Autodesk Inventor part; units mm, degrees
(part 3 of 5)
sketch "Sketch5" plane through (0, 0, 5) normal (0, 0, 1) x (1, 0, 0)
  line L0 (140, 35) -> (-140, 35) projected
  line L1 (-140, -35) -> (140, -35) projected
  line L2 (-165, 10) -> (-165, -10) projected
  line L3 (165, -10) -> (165, 10) projected
  arc A0 (87.0071, 22.2929) -> (87.7142, 22) centre (87.7142, 23) ccw
  arc A1 (87.7142, 27) -> (87.0071, 26.7071) centre (87.7142, 26) ccw
  line L4 (87.0071, 22.2929) -> (85.1, 24.2)
  line L5 (87.0071, 26.7071) -> (85.1, 24.8)
  line L6 (85.1, 24.5) -> (85.1, 24.2)
  line L7 (85.1, 24.5) -> (85.1, 24.8)
  line L8 (87.7142, 27) -> (104.4858, 27)
  line L9 (104.4858, 22) -> (87.7142, 22)
  arc A2 (105.1929, 26.7071) -> (104.4858, 27) centre (104.4858, 26) ccw
  line L10 (105.1929, 26.7071) -> (107.1, 24.8)
  line L11 (107.1, 24.5) -> (107.1, 24.8)
  line L12 (107.1, 24.5) -> (107.1, 24.2)
  arc A3 (104.4858, 22) -> (105.1929, 22.2929) centre (104.4858, 23) ccw
  line L13 (105.1929, 22.2929) -> (107.1, 24.2)
  arc A4 (87.0071, -2.5071) -> (87.7142, -2.8) centre (87.7142, -1.8) ccw
  arc A5 (87.7142, 2.2) -> (87.0071, 1.9071) centre (87.7142, 1.2) ccw
  line L14 (87.0071, -2.5071) -> (85.1, -0.6)
  line L15 (87.0071, 1.9071) -> (85.1, 0)
  line L16 (85.1, -0.3) -> (85.1, -0.6)
  line L17 (85.1, -0.3) -> (85.1, 0)
  line L18 (87.7142, 2.2) -> (104.4858, 2.2)
  line L19 (104.4858, -2.8) -> (87.7142, -2.8)
  arc A6 (105.1929, 1.9071) -> (104.4858, 2.2) centre (104.4858, 1.2) ccw
  line L20 (105.1929, 1.9071) -> (107.1, 0)
  line L21 (107.1, -0.3) -> (107.1, 0)
  line L22 (107.1, -0.3) -> (107.1, -0.6)
  arc A7 (104.4858, -2.8) -> (105.1929, -2.5071) centre (104.4858, -1.8) ccw
  line L23 (105.1929, -2.5071) -> (107.1, -0.6)
  arc A8 (85.9071, 3.0071) -> (86.2, 3.7142) centre (85.2, 3.7142) ccw
  arc A9 (81.2, 3.7142) -> (81.4929, 3.0071) centre (82.2, 3.7142) ccw
  line L24 (85.9071, 3.0071) -> (84, 1.1)
  line L25 (81.4929, 3.0071) -> (83.4, 1.1)
  line L26 (83.7, 1.1) -> (84, 1.1)
  line L27 (83.7, 1.1) -> (83.4, 1.1)
  line L28 (81.2, 3.7142) -> (81.2, 20.4858)
  line L29 (86.2, 20.4858) -> (86.2, 3.7142)
  arc A10 (81.4929, 21.1929) -> (81.2, 20.4858) centre (82.2, 20.4858) ccw
  line L30 (81.4929, 21.1929) -> (83.4, 23.1)
  line L31 (83.7, 23.1) -> (83.4, 23.1)
  line L32 (83.7, 23.1) -> (84, 23.1)
  arc A11 (86.2, 20.4858) -> (85.9071, 21.1929) centre (85.2, 20.4858) ccw
  line L33 (85.9071, 21.1929) -> (84, 23.1)
  arc A12 (85.9071, -21.7929) -> (86.2, -21.0858) centre (85.2, -21.0858) ccw
  arc A13 (81.2, -21.0858) -> (81.4929, -21.7929) centre (82.2, -21.0858) ccw
  line L34 (85.9071, -21.7929) -> (84, -23.7)
  line L35 (81.4929, -21.7929) -> (83.4, -23.7)
  line L36 (83.7, -23.7) -> (84, -23.7)
  line L37 (83.7, -23.7) -> (83.4, -23.7)
  line L38 (81.2, -21.0858) -> (81.2, -4.3142)
  line L39 (86.2, -4.3142) -> (86.2, -21.0858)
  arc A14 (81.4929, -3.6071) -> (81.2, -4.3142) centre (82.2, -4.3142) ccw
  line L40 (81.4929, -3.6071) -> (83.4, -1.7)
  line L41 (83.7, -1.7) -> (83.4, -1.7)
  line L42 (83.7, -1.7) -> (84, -1.7)
  arc A15 (86.2, -4.3142) -> (85.9071, -3.6071) centre (85.2, -4.3142) ccw
  line L43 (85.9071, -3.6071) -> (84, -1.7)
  arc A16 (110.7071, 3.0071) -> (111, 3.7142) centre (110, 3.7142) ccw
  arc A17 (106, 3.7142) -> (106.2929, 3.0071) centre (107, 3.7142) ccw
  line L44 (110.7071, 3.0071) -> (108.8, 1.1)
  line L45 (106.2929, 3.0071) -> (108.2, 1.1)
  line L46 (108.5, 1.1) -> (108.8, 1.1)
  line L47 (108.5, 1.1) -> (108.2, 1.1)
  line L48 (106, 3.7142) -> (106, 20.4858)
  line L49 (111, 20.4858) -> (111, 3.7142)
  arc A18 (106.2929, 21.1929) -> (106, 20.4858) centre (107, 20.4858) ccw
  line L50 (106.2929, 21.1929) -> (108.2, 23.1)
  line L51 (108.5, 23.1) -> (108.2, 23.1)
  line L52 (108.5, 23.1) -> (108.8, 23.1)
  arc A19 (111, 20.4858) -> (110.7071, 21.1929) centre (110, 20.4858) ccw
  line L53 (110.7071, 21.1929) -> (108.8, 23.1)
  arc A20 (110.7071, -21.7929) -> (111, -21.0858) centre (110, -21.0858) ccw
  arc A21 (106, -21.0858) -> (106.2929, -21.7929) centre (107, -21.0858) ccw
  line L54 (110.7071, -21.7929) -> (108.8, -23.7)
  line L55 (106.2929, -21.7929) -> (108.2, -23.7)
  line L56 (108.5, -23.7) -> (108.8, -23.7)
  line L57 (108.5, -23.7) -> (108.2, -23.7)
  line L58 (106, -21.0858) -> (106, -4.3142)
  line L59 (111, -4.3142) -> (111, -21.0858)
  arc A22 (106.2929, -3.6071) -> (106, -4.3142) centre (107, -4.3142) ccw
  line L60 (106.2929, -3.6071) -> (108.2, -1.7)
  line L61 (108.5, -1.7) -> (108.2, -1.7)
  line L62 (108.5, -1.7) -> (108.8, -1.7)
  arc A23 (111, -4.3142) -> (110.7071, -3.6071) centre (110, -4.3142) ccw
  line L63 (110.7071, -3.6071) -> (108.8, -1.7)
  arc A24 (87.0071, -27.3071) -> (87.7142, -27.6) centre (87.7142, -26.6) ccw
  arc A25 (87.7142, -22.6) -> (87.0071, -22.8929) centre (87.7142, -23.6) ccw
  line L64 (87.0071, -27.3071) -> (85.1, -25.4)
  line L65 (87.0071, -22.8929) -> (85.1, -24.8)
  line L66 (85.1, -25.1) -> (85.1, -25.4)
  line L67 (85.1, -25.1) -> (85.1, -24.8)
  line L68 (87.7142, -22.6) -> (104.4858, -22.6)
  line L69 (104.4858, -27.6) -> (87.7142, -27.6)
  arc A26 (105.1929, -22.8929) -> (104.4858, -22.6) centre (104.4858, -23.6) ccw
  line L70 (105.1929, -22.8929) -> (107.1, -24.8)
  line L71 (107.1, -25.1) -> (107.1, -24.8)
  line L72 (107.1, -25.1) -> (107.1, -25.4)
  arc A27 (104.4858, -27.6) -> (105.1929, -27.3071) centre (104.4858, -26.6) ccw
  line L73 (105.1929, -27.3071) -> (107.1, -25.4)
  arc A28 (40.2071, 22.2929) -> (40.9142, 22) centre (40.9142, 23) ccw
  arc A29 (40.9142, 27) -> (40.2071, 26.7071) centre (40.9142, 26) ccw
  line L74 (40.2071, 22.2929) -> (38.3, 24.2)
  line L75 (40.2071, 26.7071) -> (38.3, 24.8)
  line L76 (38.3, 24.5) -> (38.3, 24.2)
  line L77 (38.3, 24.5) -> (38.3, 24.8)
  line L78 (40.9142, 27) -> (57.6858, 27)
  line L79 (57.6858, 22) -> (40.9142, 22)
  arc A30 (58.3929, 26.7071) -> (57.6858, 27) centre (57.6858, 26) ccw
  line L80 (58.3929, 26.7071) -> (60.3, 24.8)
  line L81 (60.3, 24.5) -> (60.3, 24.8)
  line L82 (60.3, 24.5) -> (60.3, 24.2)
  arc A31 (57.6858, 22) -> (58.3929, 22.2929) centre (57.6858, 23) ccw
  line L83 (58.3929, 22.2929) -> (60.3, 24.2)
  arc A32 (40.2071, -2.5071) -> (40.9142, -2.8) centre (40.9142, -1.8) ccw
  arc A33 (40.9142, 2.2) -> (40.2071, 1.9071) centre (40.9142, 1.2) ccw
  line L84 (40.2071, -2.5071) -> (38.3, -0.6)
  line L85 (40.2071, 1.9071) -> (38.3, 0)
  line L86 (38.3, -0.3) -> (38.3, -0.6)
  line L87 (38.3, -0.3) -> (38.3, 0)
  line L88 (40.9142, 2.2) -> (57.6858, 2.2)
  line L89 (57.6858, -2.8) -> (40.9142, -2.8)
  arc A34 (58.3929, 1.9071) -> (57.6858, 2.2) centre (57.6858, 1.2) ccw
  line L90 (58.3929, 1.9071) -> (60.3, 0)
  line L91 (60.3, -0.3) -> (60.3, 0)
  line L92 (60.3, -0.3) -> (60.3, -0.6)
  arc A35 (57.6858, -2.8) -> (58.3929, -2.5071) centre (57.6858, -1.8) ccw
  line L93 (58.3929, -2.5071) -> (60.3, -0.6)
  arc A36 (39.1071, 3.0071) -> (39.4, 3.7142) centre (38.4, 3.7142) ccw
  arc A37 (34.4, 3.7142) -> (34.6929, 3.0071) centre (35.4, 3.7142) ccw
  line L94 (39.1071, 3.0071) -> (37.2, 1.1)
  line L95 (34.6929, 3.0071) -> (36.6, 1.1)
  line L96 (36.9, 1.1) -> (37.2, 1.1)
  line L97 (36.9, 1.1) -> (36.6, 1.1)
  line L98 (34.4, 3.7142) -> (34.4, 20.4858)
  line L99 (39.4, 20.4858) -> (39.4, 3.7142)
  arc A38 (34.6929, 21.1929) -> (34.4, 20.4858) centre (35.4, 20.4858) ccw
  line L100 (34.6929, 21.1929) -> (36.6, 23.1)
  line L101 (36.9, 23.1) -> (36.6, 23.1)
  line L102 (36.9, 23.1) -> (37.2, 23.1)
  arc A39 (39.4, 20.4858) -> (39.1071, 21.1929) centre (38.4, 20.4858) ccw
  line L103 (39.1071, 21.1929) -> (37.2, 23.1)
  arc A40 (39.1071, -21.7929) -> (39.4, -21.0858) centre (38.4, -21.0858) ccw
  arc A41 (34.4, -21.0858) -> (34.6929, -21.7929) centre (35.4, -21.0858) ccw
  line L104 (39.1071, -21.7929) -> (37.2, -23.7)
  line L105 (34.6929, -21.7929) -> (36.6, -23.7)
  line L106 (36.9, -23.7) -> (37.2, -23.7)
  line L107 (36.9, -23.7) -> (36.6, -23.7)
  line L108 (34.4, -21.0858) -> (34.4, -4.3142)
  line L109 (39.4, -4.3142) -> (39.4, -21.0858)
  arc A42 (34.6929, -3.6071) -> (34.4, -4.3142) centre (35.4, -4.3142) ccw
  line L110 (34.6929, -3.6071) -> (36.6, -1.7)
  line L111 (36.9, -1.7) -> (36.6, -1.7)
  line L112 (36.9, -1.7) -> (37.2, -1.7)
  arc A43 (39.4, -4.3142) -> (39.1071, -3.6071) centre (38.4, -4.3142) ccw
  line L113 (39.1071, -3.6071) -> (37.2, -1.7)
  arc A44 (63.9071, 3.0071) -> (64.2, 3.7142) centre (63.2, 3.7142) ccw
  arc A45 (59.2, 3.7142) -> (59.4929, 3.0071) centre (60.2, 3.7142) ccw
  line L114 (63.9071, 3.0071) -> (62, 1.1)
  line L115 (59.4929, 3.0071) -> (61.4, 1.1)
  line L116 (61.7, 1.1) -> (62, 1.1)
  line L117 (61.7, 1.1) -> (61.4, 1.1)
  line L118 (59.2, 3.7142) -> (59.2, 20.4858)
  line L119 (64.2, 20.4858) -> (64.2, 3.7142)
  arc A46 (59.4929, 21.1929) -> (59.2, 20.4858) centre (60.2, 20.4858) ccw
  line L120 (59.4929, 21.1929) -> (61.4, 23.1)
  line L121 (61.7, 23.1) -> (61.4, 23.1)
  line L122 (61.7, 23.1) -> (62, 23.1)
  arc A47 (64.2, 20.4858) -> (63.9071, 21.1929) centre (63.2, 20.4858) ccw
  line L123 (63.9071, 21.1929) -> (62, 23.1)
  arc A48 (63.9071, -21.7929) -> (64.2, -21.0858) centre (63.2, -21.0858) ccw
  arc A49 (59.2, -21.0858) -> (59.4929, -21.7929) centre (60.2, -21.0858) ccw
  line L124 (63.9071, -21.7929) -> (62, -23.7)
  line L125 (59.4929, -21.7929) -> (61.4, -23.7)
  line L126 (61.7, -23.7) -> (62, -23.7)
  line L127 (61.7, -23.7) -> (61.4, -23.7)
  line L128 (59.2, -21.0858) -> (59.2, -4.3142)
  line L129 (64.2, -4.3142) -> (64.2, -21.0858)
  arc A50 (59.4929, -3.6071) -> (59.2, -4.3142) centre (60.2, -4.3142) ccw
  line L130 (59.4929, -3.6071) -> (61.4, -1.7)
  line L131 (61.7, -1.7) -> (61.4, -1.7)
  line L132 (61.7, -1.7) -> (62, -1.7)
  arc A51 (64.2, -4.3142) -> (63.9071, -3.6071) centre (63.2, -4.3142) ccw
  line L133 (63.9071, -3.6071) -> (62, -1.7)
  arc A52 (40.2071, -27.3071) -> (40.9142, -27.6) centre (40.9142, -26.6) ccw
  arc A53 (40.9142, -22.6) -> (40.2071, -22.8929) centre (40.9142, -23.6) ccw
  line L134 (40.2071, -27.3071) -> (38.3, -25.4)
  line L135 (40.2071, -22.8929) -> (38.3, -24.8)
  line L136 (38.3, -25.1) -> (38.3, -25.4)
  line L137 (38.3, -25.1) -> (38.3, -24.8)
  line L138 (40.9142, -22.6) -> (57.6858, -22.6)
  line L139 (57.6858, -27.6) -> (40.9142, -27.6)
  arc A54 (58.3929, -22.8929) -> (57.6858, -22.6) centre (57.6858, -23.6) ccw
  line L140 (58.3929, -22.8929) -> (60.3, -24.8)
  line L141 (60.3, -25.1) -> (60.3, -24.8)
  line L142 (60.3, -25.1) -> (60.3, -25.4)
  arc A55 (57.6858, -27.6) -> (58.3929, -27.3071) centre (57.6858, -26.6) ccw
  line L143 (58.3929, -27.3071) -> (60.3, -25.4)
  arc A56 (2.9071, 22.2929) -> (3.6142, 22) centre (3.6142, 23) ccw
  arc A57 (3.6142, 27) -> (2.9071, 26.7071) centre (3.6142, 26) ccw
  line L144 (2.9071, 22.2929) -> (1, 24.2)
  line L145 (2.9071, 26.7071) -> (1, 24.8)
  line L146 (1, 24.5) -> (1, 24.2)
  line L147 (1, 24.5) -> (1, 24.8)
  line L148 (3.6142, 27) -> (20.3858, 27)
  line L149 (20.3858, 22) -> (3.6142, 22)
  arc A58 (21.0929, 26.7071) -> (20.3858, 27) centre (20.3858, 26) ccw
  line L150 (21.0929, 26.7071) -> (23, 24.8)
  line L151 (23, 24.5) -> (23, 24.8)
  line L152 (23, 24.5) -> (23, 24.2)
  arc A59 (20.3858, 22) -> (21.0929, 22.2929) centre (20.3858, 23) ccw
  line L153 (21.0929, 22.2929) -> (23, 24.2)
  arc A60 (2.9071, -2.5071) -> (3.6142, -2.8) centre (3.6142, -1.8) ccw
  arc A61 (3.6142, 2.2) -> (2.9071, 1.9071) centre (3.6142, 1.2) ccw
  line L154 (2.9071, -2.5071) -> (1, -0.6)
  line L155 (2.9071, 1.9071) -> (1, 0)
  line L156 (1, -0.3) -> (1, -0.6)
  line L157 (1, -0.3) -> (1, 0)
  line L158 (3.6142, 2.2) -> (20.3858, 2.2)
  line L159 (20.3858, -2.8) -> (3.6142, -2.8)
  arc A62 (21.0929, 1.9071) -> (20.3858, 2.2) centre (20.3858, 1.2) ccw
  line L160 (21.0929, 1.9071) -> (23, 0)
  line L161 (23, -0.3) -> (23, 0)
  line L162 (23, -0.3) -> (23, -0.6)
  arc A63 (20.3858, -2.8) -> (21.0929, -2.5071) centre (20.3858, -1.8) ccw
  line L163 (21.0929, -2.5071) -> (23, -0.6)
  arc A64 (1.8071, 3.0071) -> (2.1, 3.7142) centre (1.1, 3.7142) ccw
  arc A65 (-2.9, 3.7142) -> (-2.6071, 3.0071) centre (-1.9, 3.7142) ccw
  line L164 (1.8071, 3.0071) -> (-0.1, 1.1)
  line L165 (-2.6071, 3.0071) -> (-0.7, 1.1)
  line L166 (-0.4, 1.1) -> (-0.1, 1.1)
  line L167 (-0.4, 1.1) -> (-0.7, 1.1)
  line L168 (-2.9, 3.7142) -> (-2.9, 20.4858)
  line L169 (2.1, 20.4858) -> (2.1, 3.7142)
  arc A66 (-2.6071, 21.1929) -> (-2.9, 20.4858) centre (-1.9, 20.4858) ccw
  line L170 (-2.6071, 21.1929) -> (-0.7, 23.1)
  line L171 (-0.4, 23.1) -> (-0.7, 23.1)
  line L172 (-0.4, 23.1) -> (-0.1, 23.1)
  arc A67 (2.1, 20.4858) -> (1.8071, 21.1929) centre (1.1, 20.4858) ccw
  line L173 (1.8071, 21.1929) -> (-0.1, 23.1)
  arc A68 (1.8071, -21.7929) -> (2.1, -21.0858) centre (1.1, -21.0858) ccw
  arc A69 (-2.9, -21.0858) -> (-2.6071, -21.7929) centre (-1.9, -21.0858) ccw
  line L174 (1.8071, -21.7929) -> (-0.1, -23.7)
  line L175 (-2.6071, -21.7929) -> (-0.7, -23.7)
  line L176 (-0.4, -23.7) -> (-0.1, -23.7)
  line L177 (-0.4, -23.7) -> (-0.7, -23.7)
  line L178 (-2.9, -21.0858) -> (-2.9, -4.3142)
  line L179 (2.1, -4.3142) -> (2.1, -21.0858)
  arc A70 (-2.6071, -3.6071) -> (-2.9, -4.3142) centre (-1.9, -4.3142) ccw
  line L180 (-2.6071, -3.6071) -> (-0.7, -1.7)
  line L181 (-0.4, -1.7) -> (-0.7, -1.7)
  line L182 (-0.4, -1.7) -> (-0.1, -1.7)
  arc A71 (2.1, -4.3142) -> (1.8071, -3.6071) centre (1.1, -4.3142) ccw
  line L183 (1.8071, -3.6071) -> (-0.1, -1.7)
  arc A72 (26.6071, 3.0071) -> (26.9, 3.7142) centre (25.9, 3.7142) ccw
  arc A73 (21.9, 3.7142) -> (22.1929, 3.0071) centre (22.9, 3.7142) ccw
  line L184 (26.6071, 3.0071) -> (24.7, 1.1)
  line L185 (22.1929, 3.0071) -> (24.1, 1.1)
  line L186 (24.4, 1.1) -> (24.7, 1.1)
  line L187 (24.4, 1.1) -> (24.1, 1.1)
  line L188 (21.9, 3.7142) -> (21.9, 20.4858)
  line L189 (26.9, 20.4858) -> (26.9, 3.7142)
  arc A74 (22.1929, 21.1929) -> (21.9, 20.4858) centre (22.9, 20.4858) ccw
  line L190 (22.1929, 21.1929) -> (24.1, 23.1)
  line L191 (24.4, 23.1) -> (24.1, 23.1)
  line L192 (24.4, 23.1) -> (24.7, 23.1)
  arc A75 (26.9, 20.4858) -> (26.6071, 21.1929) centre (25.9, 20.4858) ccw
  line L193 (26.6071, 21.1929) -> (24.7, 23.1)
  arc A76 (26.6071, -21.7929) -> (26.9, -21.0858) centre (25.9, -21.0858) ccw
  arc A77 (21.9, -21.0858) -> (22.1929, -21.7929) centre (22.9, -21.0858) ccw
  line L194 (26.6071, -21.7929) -> (24.7, -23.7)
  line L195 (22.1929, -21.7929) -> (24.1, -23.7)
  line L196 (24.4, -23.7) -> (24.7, -23.7)
  line L197 (24.4, -23.7) -> (24.1, -23.7)
  line L198 (21.9, -21.0858) -> (21.9, -4.3142)
  line L199 (26.9, -4.3142) -> (26.9, -21.0858)
  arc A78 (22.1929, -3.6071) -> (21.9, -4.3142) centre (22.9, -4.3142) ccw
  line L200 (22.1929, -3.6071) -> (24.1, -1.7)
  line L201 (24.4, -1.7) -> (24.1, -1.7)
  line L202 (24.4, -1.7) -> (24.7, -1.7)
  arc A79 (26.9, -4.3142) -> (26.6071, -3.6071) centre (25.9, -4.3142) ccw
  line L203 (26.6071, -3.6071) -> (24.7, -1.7)
  arc A80 (2.9071, -27.3071) -> (3.6142, -27.6) centre (3.6142, -26.6) ccw
  arc A81 (3.6142, -22.6) -> (2.9071, -22.8929) centre (3.6142, -23.6) ccw
  line L204 (2.9071, -27.3071) -> (1, -25.4)
  line L205 (2.9071, -22.8929) -> (1, -24.8)
  line L206 (1, -25.1) -> (1, -25.4)
  line L207 (1, -25.1) -> (1, -24.8)
  line L208 (3.6142, -22.6) -> (20.3858, -22.6)
  line L209 (20.3858, -27.6) -> (3.6142, -27.6)
  arc A82 (21.0929, -22.8929) -> (20.3858, -22.6) centre (20.3858, -23.6) ccw
  line L210 (21.0929, -22.8929) -> (23, -24.8)
  line L211 (23, -25.1) -> (23, -24.8)
  line L212 (23, -25.1) -> (23, -25.4)
  arc A83 (20.3858, -27.6) -> (21.0929, -27.3071) centre (20.3858, -26.6) ccw
  line L213 (21.0929, -27.3071) -> (23, -25.4)
  arc A84 (-43.8929, 22.2929) -> (-43.1858, 22) centre (-43.1858, 23) ccw
  arc A85 (-43.1858, 27) -> (-43.8929, 26.7071) centre (-43.1858, 26) ccw
  line L214 (-43.8929, 22.2929) -> (-45.8, 24.2)
  line L215 (-43.8929, 26.7071) -> (-45.8, 24.8)
  line L216 (-45.8, 24.5) -> (-45.8, 24.2)
  line L217 (-45.8, 24.5) -> (-45.8, 24.8)
  line L218 (-43.1858, 27) -> (-26.4142, 27)
  line L219 (-26.4142, 22) -> (-43.1858, 22)
  arc A86 (-25.7071, 26.7071) -> (-26.4142, 27) centre (-26.4142, 26) ccw
  line L220 (-25.7071, 26.7071) -> (-23.8, 24.8)
  line L221 (-23.8, 24.5) -> (-23.8, 24.8)
  line L222 (-23.8, 24.5) -> (-23.8, 24.2)
  arc A87 (-26.4142, 22) -> (-25.7071, 22.2929) centre (-26.4142, 23) ccw
  line L223 (-25.7071, 22.2929) -> (-23.8, 24.2)
  arc A88 (-43.8929, -2.5071) -> (-43.1858, -2.8) centre (-43.1858, -1.8) ccw
  arc A89 (-43.1858, 2.2) -> (-43.8929, 1.9071) centre (-43.1858, 1.2) ccw
  line L224 (-43.8929, -2.5071) -> (-45.8, -0.6)
  line L225 (-43.8929, 1.9071) -> (-45.8, 0)
  line L226 (-45.8, -0.3) -> (-45.8, -0.6)
  line L227 (-45.8, -0.3) -> (-45.8, 0)
  line L228 (-43.1858, 2.2) -> (-26.4142, 2.2)
  line L229 (-26.4142, -2.8) -> (-43.1858, -2.8)
  arc A90 (-25.7071, 1.9071) -> (-26.4142, 2.2) centre (-26.4142, 1.2) ccw
  line L230 (-25.7071, 1.9071) -> (-23.8, 0)
  line L231 (-23.8, -0.3) -> (-23.8, 0)
  line L232 (-23.8, -0.3) -> (-23.8, -0.6)
  arc A91 (-26.4142, -2.8) -> (-25.7071, -2.5071) centre (-26.4142, -1.8) ccw
  line L233 (-25.7071, -2.5071) -> (-23.8, -0.6)
  arc A92 (-44.9929, 3.0071) -> (-44.7, 3.7142) centre (-45.7, 3.7142) ccw
  arc A93 (-49.7, 3.7142) -> (-49.4071, 3.0071) centre (-48.7, 3.7142) ccw
  line L234 (-44.9929, 3.0071) -> (-46.9, 1.1)
  line L235 (-49.4071, 3.0071) -> (-47.5, 1.1)
  line L236 (-47.2, 1.1) -> (-46.9, 1.1)
  line L237 (-47.2, 1.1) -> (-47.5, 1.1)
  line L238 (-49.7, 3.7142) -> (-49.7, 20.4858)
  line L239 (-44.7, 20.4858) -> (-44.7, 3.7142)
  arc A94 (-49.4071, 21.1929) -> (-49.7, 20.4858) centre (-48.7, 20.4858) ccw
  line L240 (-49.4071, 21.1929) -> (-47.5, 23.1)
  line L241 (-47.2, 23.1) -> (-47.5, 23.1)
  line L242 (-47.2, 23.1) -> (-46.9, 23.1)
  arc A95 (-44.7, 20.4858) -> (-44.9929, 21.1929) centre (-45.7, 20.4858) ccw
  line L243 (-44.9929, 21.1929) -> (-46.9, 23.1)
  arc A96 (-44.9929, -21.7929) -> (-44.7, -21.0858) centre (-45.7, -21.0858) ccw
  arc A97 (-49.7, -21.0858) -> (-49.4071, -21.7929) centre (-48.7, -21.0858) ccw
  line L244 (-44.9929, -21.7929) -> (-46.9, -23.7)
  line L245 (-49.4071, -21.7929) -> (-47.5, -23.7)
  line L246 (-47.2, -23.7) -> (-46.9, -23.7)
  line L247 (-47.2, -23.7) -> (-47.5, -23.7)
  line L248 (-49.7, -21.0858) -> (-49.7, -4.3142)
  line L249 (-44.7, -4.3142) -> (-44.7, -21.0858)
  arc A98 (-49.4071, -3.6071) -> (-49.7, -4.3142) centre (-48.7, -4.3142) ccw
  line L250 (-49.4071, -3.6071) -> (-47.5, -1.7)
  line L251 (-47.2, -1.7) -> (-47.5, -1.7)
  line L252 (-47.2, -1.7) -> (-46.9, -1.7)
  arc A99 (-44.7, -4.3142) -> (-44.9929, -3.6071) centre (-45.7, -4.3142) ccw
  line L253 (-44.9929, -3.6071) -> (-46.9, -1.7)
  arc A100 (-20.1929, 3.0071) -> (-19.9, 3.7142) centre (-20.9, 3.7142) ccw
  arc A101 (-24.9, 3.7142) -> (-24.6071, 3.0071) centre (-23.9, 3.7142) ccw
  line L254 (-20.1929, 3.0071) -> (-22.1, 1.1)
  line L255 (-24.6071, 3.0071) -> (-22.7, 1.1)
  line L256 (-22.4, 1.1) -> (-22.1, 1.1)
  line L257 (-22.4, 1.1) -> (-22.7, 1.1)
  line L258 (-24.9, 3.7142) -> (-24.9, 20.4858)
  line L259 (-19.9, 20.4858) -> (-19.9, 3.7142)
  arc A102 (-24.6071, 21.1929) -> (-24.9, 20.4858) centre (-23.9, 20.4858) ccw
  line L260 (-24.6071, 21.1929) -> (-22.7, 23.1)
  line L261 (-22.4, 23.1) -> (-22.7, 23.1)
  line L262 (-22.4, 23.1) -> (-22.1, 23.1)
  arc A103 (-19.9, 20.4858) -> (-20.1929, 21.1929) centre (-20.9, 20.4858) ccw
  line L263 (-20.1929, 21.1929) -> (-22.1, 23.1)
  arc A104 (-20.1929, -21.7929) -> (-19.9, -21.0858) centre (-20.9, -21.0858) ccw
  arc A105 (-24.9, -21.0858) -> (-24.6071, -21.7929) centre (-23.9, -21.0858) ccw
  line L264 (-20.1929, -21.7929) -> (-22.1, -23.7)
  line L265 (-24.6071, -21.7929) -> (-22.7, -23.7)
  line L266 (-22.4, -23.7) -> (-22.1, -23.7)
  line L267 (-22.4, -23.7) -> (-22.7, -23.7)
  line L268 (-24.9, -21.0858) -> (-24.9, -4.3142)
  line L269 (-19.9, -4.3142) -> (-19.9, -21.0858)
  arc A106 (-24.6071, -3.6071) -> (-24.9, -4.3142) centre (-23.9, -4.3142) ccw
  line L270 (-24.6071, -3.6071) -> (-22.7, -1.7)
  line L271 (-22.4, -1.7) -> (-22.7, -1.7)
  line L272 (-22.4, -1.7) -> (-22.1, -1.7)
  arc A107 (-19.9, -4.3142) -> (-20.1929, -3.6071) centre (-20.9, -4.3142) ccw
  line L273 (-20.1929, -3.6071) -> (-22.1, -1.7)
  arc A108 (-43.8929, -27.3071) -> (-43.1858, -27.6) centre (-43.1858, -26.6) ccw
  arc A109 (-43.1858, -22.6) -> (-43.8929, -22.8929) centre (-43.1858, -23.6) ccw
  line L274 (-43.8929, -27.3071) -> (-45.8, -25.4)
  line L275 (-43.8929, -22.8929) -> (-45.8, -24.8)
  line L276 (-45.8, -25.1) -> (-45.8, -25.4)
  line L277 (-45.8, -25.1) -> (-45.8, -24.8)
  line L278 (-43.1858, -22.6) -> (-26.4142, -22.6)
  line L279 (-26.4142, -27.6) -> (-43.1858, -27.6)
  arc A110 (-25.7071, -22.8929) -> (-26.4142, -22.6) centre (-26.4142, -23.6) ccw
  line L280 (-25.7071, -22.8929) -> (-23.8, -24.8)
  line L281 (-23.8, -25.1) -> (-23.8, -24.8)
  line L282 (-23.8, -25.1) -> (-23.8, -25.4)
  arc A111 (-26.4142, -27.6) -> (-25.7071, -27.3071) centre (-26.4142, -26.6) ccw
  line L283 (-25.7071, -27.3071) -> (-23.8, -25.4)
  arc A112 (-81.1929, 22.2929) -> (-80.4858, 22) centre (-80.4858, 23) ccw
  arc A113 (-80.4858, 27) -> (-81.1929, 26.7071) centre (-80.4858, 26) ccw
  line L284 (-81.1929, 22.2929) -> (-83.1, 24.2)
  line L285 (-81.1929, 26.7071) -> (-83.1, 24.8)
  line L286 (-83.1, 24.5) -> (-83.1, 24.2)
  line L287 (-83.1, 24.5) -> (-83.1, 24.8)
  line L288 (-80.4858, 27) -> (-63.7142, 27)
  line L289 (-63.7142, 22) -> (-80.4858, 22)
  arc A114 (-63.0071, 26.7071) -> (-63.7142, 27) centre (-63.7142, 26) ccw
  line L290 (-63.0071, 26.7071) -> (-61.1, 24.8)
  line L291 (-61.1, 24.5) -> (-61.1, 24.8)
  line L292 (-61.1, 24.5) -> (-61.1, 24.2)
  arc A115 (-63.7142, 22) -> (-63.0071, 22.2929) centre (-63.7142, 23) ccw
  line L293 (-63.0071, 22.2929) -> (-61.1, 24.2)
  arc A116 (-81.1929, -2.5071) -> (-80.4858, -2.8) centre (-80.4858, -1.8) ccw
  arc A117 (-80.4858, 2.2) -> (-81.1929, 1.9071) centre (-80.4858, 1.2) ccw
  line L294 (-81.1929, -2.5071) -> (-83.1, -0.6)
  line L295 (-81.1929, 1.9071) -> (-83.1, 0)
  line L296 (-83.1, -0.3) -> (-83.1, -0.6)
  line L297 (-83.1, -0.3) -> (-83.1, 0)
  line L298 (-80.4858, 2.2) -> (-63.7142, 2.2)
  line L299 (-63.7142, -2.8) -> (-80.4858, -2.8)
  arc A118 (-63.0071, 1.9071) -> (-63.7142, 2.2) centre (-63.7142, 1.2) ccw
  line L300 (-63.0071, 1.9071) -> (-61.1, 0)
  line L301 (-61.1, -0.3) -> (-61.1, 0)
  line L302 (-61.1, -0.3) -> (-61.1, -0.6)
  arc A119 (-63.7142, -2.8) -> (-63.0071, -2.5071) centre (-63.7142, -1.8) ccw
  line L303 (-63.0071, -2.5071) -> (-61.1, -0.6)
  arc A120 (-82.2929, 3.0071) -> (-82, 3.7142) centre (-83, 3.7142) ccw
  arc A121 (-87, 3.7142) -> (-86.7071, 3.0071) centre (-86, 3.7142) ccw
  line L304 (-82.2929, 3.0071) -> (-84.2, 1.1)
  line L305 (-86.7071, 3.0071) -> (-84.8, 1.1)
  line L306 (-84.5, 1.1) -> (-84.2, 1.1)
  line L307 (-84.5, 1.1) -> (-84.8, 1.1)
  line L308 (-87, 3.7142) -> (-87, 20.4858)
  line L309 (-82, 20.4858) -> (-82, 3.7142)
  arc A122 (-86.7071, 21.1929) -> (-87, 20.4858) centre (-86, 20.4858) ccw
  line L310 (-86.7071, 21.1929) -> (-84.8, 23.1)
  line L311 (-84.5, 23.1) -> (-84.8, 23.1)
  line L312 (-84.5, 23.1) -> (-84.2, 23.1)
  arc A123 (-82, 20.4858) -> (-82.2929, 21.1929) centre (-83, 20.4858) ccw
  line L313 (-82.2929, 21.1929) -> (-84.2, 23.1)
  arc A124 (-82.2929, -21.7929) -> (-82, -21.0858) centre (-83, -21.0858) ccw
  arc A125 (-87, -21.0858) -> (-86.7071, -21.7929) centre (-86, -21.0858) ccw
  line L314 (-82.2929, -21.7929) -> (-84.2, -23.7)
  line L315 (-86.7071, -21.7929) -> (-84.8, -23.7)
  line L316 (-84.5, -23.7) -> (-84.2, -23.7)
  line L317 (-84.5, -23.7) -> (-84.8, -23.7)
  line L318 (-87, -21.0858) -> (-87, -4.3142)
  line L319 (-82, -4.3142) -> (-82, -21.0858)
  arc A126 (-86.7071, -3.6071) -> (-87, -4.3142) centre (-86, -4.3142) ccw
  line L320 (-86.7071, -3.6071) -> (-84.8, -1.7)
  line L321 (-84.5, -1.7) -> (-84.8, -1.7)
  line L322 (-84.5, -1.7) -> (-84.2, -1.7)
  arc A127 (-82, -4.3142) -> (-82.2929, -3.6071) centre (-83, -4.3142) ccw
  line L323 (-82.2929, -3.6071) -> (-84.2, -1.7)
  arc A128 (-57.4929, 3.0071) -> (-57.2, 3.7142) centre (-58.2, 3.7142) ccw
  arc A129 (-62.2, 3.7142) -> (-61.9071, 3.0071) centre (-61.2, 3.7142) ccw
  line L324 (-57.4929, 3.0071) -> (-59.4, 1.1)
  line L325 (-61.9071, 3.0071) -> (-60, 1.1)
  line L326 (-59.7, 1.1) -> (-59.4, 1.1)
  line L327 (-59.7, 1.1) -> (-60, 1.1)
  line L328 (-62.2, 3.7142) -> (-62.2, 20.4858)
  line L329 (-57.2, 20.4858) -> (-57.2, 3.7142)
  arc A130 (-61.9071, 21.1929) -> (-62.2, 20.4858) centre (-61.2, 20.4858) ccw
  line L330 (-61.9071, 21.1929) -> (-60, 23.1)
  line L331 (-59.7, 23.1) -> (-60, 23.1)
  line L332 (-59.7, 23.1) -> (-59.4, 23.1)
  arc A131 (-57.2, 20.4858) -> (-57.4929, 21.1929) centre (-58.2, 20.4858) ccw
  line L333 (-57.4929, 21.1929) -> (-59.4, 23.1)
  arc A132 (-57.4929, -21.7929) -> (-57.2, -21.0858) centre (-58.2, -21.0858) ccw
  arc A133 (-62.2, -21.0858) -> (-61.9071, -21.7929) centre (-61.2, -21.0858) ccw
  line L334 (-57.4929, -21.7929) -> (-59.4, -23.7)
  line L335 (-61.9071, -21.7929) -> (-60, -23.7)
  line L336 (-59.7, -23.7) -> (-59.4, -23.7)
  line L337 (-59.7, -23.7) -> (-60, -23.7)
  line L338 (-62.2, -21.0858) -> (-62.2, -4.3142)
  line L339 (-57.2, -4.3142) -> (-57.2, -21.0858)
  arc A134 (-61.9071, -3.6071) -> (-62.2, -4.3142) centre (-61.2, -4.3142) ccw
  line L340 (-61.9071, -3.6071) -> (-60, -1.7)
  line L341 (-59.7, -1.7) -> (-60, -1.7)
  line L342 (-59.7, -1.7) -> (-59.4, -1.7)
  arc A135 (-57.2, -4.3142) -> (-57.4929, -3.6071) centre (-58.2, -4.3142) ccw
  line L343 (-57.4929, -3.6071) -> (-59.4, -1.7)
  arc A136 (-81.1929, -27.3071) -> (-80.4858, -27.6) centre (-80.4858, -26.6) ccw
  arc A137 (-80.4858, -22.6) -> (-81.1929, -22.8929) centre (-80.4858, -23.6) ccw
  line L344 (-81.1929, -27.3071) -> (-83.1, -25.4)
  line L345 (-81.1929, -22.8929) -> (-83.1, -24.8)
  line L346 (-83.1, -25.1) -> (-83.1, -25.4)
  line L347 (-83.1, -25.1) -> (-83.1, -24.8)
  line L348 (-80.4858, -22.6) -> (-63.7142, -22.6)
  line L349 (-63.7142, -27.6) -> (-80.4858, -27.6)
  arc A138 (-63.0071, -22.8929) -> (-63.7142, -22.6) centre (-63.7142, -23.6) ccw
  line L350 (-63.0071, -22.8929) -> (-61.1, -24.8)
  line L351 (-61.1, -25.1) -> (-61.1, -24.8)
  line L352 (-61.1, -25.1) -> (-61.1, -25.4)
  arc A139 (-63.7142, -27.6) -> (-63.0071, -27.3071) centre (-63.7142, -26.6) ccw
  line L353 (-63.0071, -27.3071) -> (-61.1, -25.4)
  arc A140 (124.3071, 22.2929) -> (125.0142, 22) centre (125.0142, 23) ccw
  arc A141 (125.0142, 27) -> (124.3071, 26.7071) centre (125.0142, 26) ccw
  line L354 (124.3071, 22.2929) -> (122.4, 24.2)
  line L355 (124.3071, 26.7071) -> (122.4, 24.8)
  line L356 (122.4, 24.5) -> (122.4, 24.2)
  line L357 (122.4, 24.5) -> (122.4, 24.8)
  line L358 (125.0142, 27) -> (141.7858, 27)
  line L359 (141.7858, 22) -> (125.0142, 22)
  arc A142 (142.4929, 26.7071) -> (141.7858, 27) centre (141.7858, 26) ccw
  line L360 (142.4929, 26.7071) -> (144.4, 24.8)
  line L361 (144.4, 24.5) -> (144.4, 24.8)
  line L362 (144.4, 24.5) -> (144.4, 24.2)
  arc A143 (141.7858, 22) -> (142.4929, 22.2929) centre (141.7858, 23) ccw
  line L363 (142.4929, 22.2929) -> (144.4, 24.2)
  arc A144 (124.3071, -2.5071) -> (125.0142, -2.8) centre (125.0142, -1.8) ccw
  arc A145 (125.0142, 2.2) -> (124.3071, 1.9071) centre (125.0142, 1.2) ccw
  line L364 (124.3071, -2.5071) -> (122.4, -0.6)
  line L365 (124.3071, 1.9071) -> (122.4, 0)
  line L366 (122.4, -0.3) -> (122.4, -0.6)
  line L367 (122.4, -0.3) -> (122.4, 0)
  line L368 (125.0142, 2.2) -> (141.7858, 2.2)
  line L369 (141.7858, -2.8) -> (125.0142, -2.8)
  arc A146 (142.4929, 1.9071) -> (141.7858, 2.2) centre (141.7858, 1.2) ccw
  line L370 (142.4929, 1.9071) -> (144.4, 0)
  line L371 (144.4, -0.3) -> (144.4, 0)
  line L372 (144.4, -0.3) -> (144.4, -0.6)
  arc A147 (141.7858, -2.8) -> (142.4929, -2.5071) centre (141.7858, -1.8) ccw
  line L373 (142.4929, -2.5071) -> (144.4, -0.6)
  arc A148 (123.2071, 3.0071) -> (123.5, 3.7142) centre (122.5, 3.7142) ccw
  arc A149 (118.5, 3.7142) -> (118.7929, 3.0071) centre (119.5, 3.7142) ccw
  line L374 (123.2071, 3.0071) -> (121.3, 1.1)
  line L375 (118.7929, 3.0071) -> (120.7, 1.1)
  line L376 (121, 1.1) -> (121.3, 1.1)
  line L377 (121, 1.1) -> (120.7, 1.1)
  line L378 (118.5, 3.7142) -> (118.5, 20.4858)
  line L379 (123.5, 20.4858) -> (123.5, 3.7142)
  arc A150 (118.7929, 21.1929) -> (118.5, 20.4858) centre (119.5, 20.4858) ccw
  line L380 (118.7929, 21.1929) -> (120.7, 23.1)
  line L381 (121, 23.1) -> (120.7, 23.1)
  line L382 (121, 23.1) -> (121.3, 23.1)
  arc A151 (123.5, 20.4858) -> (123.2071, 21.1929) centre (122.5, 20.4858) ccw
  line L383 (123.2071, 21.1929) -> (121.3, 23.1)
  arc A152 (123.2071, -21.7929) -> (123.5, -21.0858) centre (122.5, -21.0858) ccw
  arc A153 (118.5, -21.0858) -> (118.7929, -21.7929) centre (119.5, -21.0858) ccw
  line L384 (123.2071, -21.7929) -> (121.3, -23.7)
  line L385 (118.7929, -21.7929) -> (120.7, -23.7)
  line L386 (121, -23.7) -> (121.3, -23.7)
  line L387 (121, -23.7) -> (120.7, -23.7)
  line L388 (118.5, -21.0858) -> (118.5, -4.3142)
  line L389 (123.5, -4.3142) -> (123.5, -21.0858)
  arc A154 (118.7929, -3.6071) -> (118.5, -4.3142) centre (119.5, -4.3142) ccw
  line L390 (118.7929, -3.6071) -> (120.7, -1.7)
  line L391 (121, -1.7) -> (120.7, -1.7)
  line L392 (121, -1.7) -> (121.3, -1.7)
  arc A155 (123.5, -4.3142) -> (123.2071, -3.6071) centre (122.5, -4.3142) ccw
  line L393 (123.2071, -3.6071) -> (121.3, -1.7)
  arc A156 (148.0071, 3.0071) -> (148.3, 3.7142) centre (147.3, 3.7142) ccw
  arc A157 (143.3, 3.7142) -> (143.5929, 3.0071) centre (144.3, 3.7142) ccw
  line L394 (148.0071, 3.0071) -> (146.1, 1.1)
  line L395 (143.5929, 3.0071) -> (145.5, 1.1)
  line L396 (145.8, 1.1) -> (146.1, 1.1)
  line L397 (145.8, 1.1) -> (145.5, 1.1)
  line L398 (143.3, 3.7142) -> (143.3, 20.4858)
  line L399 (148.3, 20.4858) -> (148.3, 3.7142)
  arc A158 (143.5929, 21.1929) -> (143.3, 20.4858) centre (144.3, 20.4858) ccw
  line L400 (143.5929, 21.1929) -> (145.5, 23.1)
  line L401 (145.8, 23.1) -> (145.5, 23.1)
  line L402 (145.8, 23.1) -> (146.1, 23.1)
  arc A159 (148.3, 20.4858) -> (148.0071, 21.1929) centre (147.3, 20.4858) ccw
  line L403 (148.0071, 21.1929) -> (146.1, 23.1)
  arc A160 (148.0071, -21.7929) -> (148.3, -21.0858) centre (147.3, -21.0858) ccw
  arc A161 (143.3, -21.0858) -> (143.5929, -21.7929) centre (144.3, -21.0858) ccw
  line L404 (148.0071, -21.7929) -> (146.1, -23.7)
  line L405 (143.5929, -21.7929) -> (145.5, -23.7)
  line L406 (145.8, -23.7) -> (146.1, -23.7)
  line L407 (145.8, -23.7) -> (145.5, -23.7)
  line L408 (143.3, -21.0858) -> (143.3, -4.3142)
  line L409 (148.3, -4.3142) -> (148.3, -21.0858)
  arc A162 (143.5929, -3.6071) -> (143.3, -4.3142) centre (144.3, -4.3142) ccw
  line L410 (143.5929, -3.6071) -> (145.5, -1.7)
  line L411 (145.8, -1.7) -> (145.5, -1.7)
  line L412 (145.8, -1.7) -> (146.1, -1.7)
  arc A163 (148.3, -4.3142) -> (148.0071, -3.6071) centre (147.3, -4.3142) ccw
  line L413 (148.0071, -3.6071) -> (146.1, -1.7)
  arc A164 (124.3071, -27.3071) -> (125.0142, -27.6) centre (125.0142, -26.6) ccw
  arc A165 (125.0142, -22.6) -> (124.3071, -22.8929) centre (125.0142, -23.6) ccw
  line L414 (124.3071, -27.3071) -> (122.4, -25.4)
  line L415 (124.3071, -22.8929) -> (122.4, -24.8)
  line L416 (122.4, -25.1) -> (122.4, -25.4)
  line L417 (122.4, -25.1) -> (122.4, -24.8)
  line L418 (125.0142, -22.6) -> (141.7858, -22.6)
  line L419 (141.7858, -27.6) -> (125.0142, -27.6)
  arc A166 (142.4929, -22.8929) -> (141.7858, -22.6) centre (141.7858, -23.6) ccw
  line L420 (142.4929, -22.8929) -> (144.4, -24.8)
  line L421 (144.4, -25.1) -> (144.4, -24.8)
  line L422 (144.4, -25.1) -> (144.4, -25.4)
  arc A167 (141.7858, -27.6) -> (142.4929, -27.3071) centre (141.7858, -26.6) ccw
  line L423 (142.4929, -27.3071) -> (144.4, -25.4)
  line L424 (-11.9, 11) -> (-10.9, 11)
  line L425 (-10.9, 11) -> (-8.9, 9)
  line L426 (-8.9, 9) -> (-8.9, 8)
  line L427 (-8.9, 8) -> (-10.9, 6)
  line L428 (-10.9, 6) -> (-11.9, 6)
  line L429 (-11.9, 6) -> (-13.9, 8)
  line L430 (-13.9, 8) -> (-13.9, 9)
  line L431 (-13.9, 9) -> (-11.9, 11)
  line L432 (-11.9, -9) -> (-10.9, -9)
  line L433 (-10.9, -9) -> (-8.9, -11)
  line L434 (-8.9, -11) -> (-8.9, -12)
  line L435 (-8.9, -12) -> (-10.9, -14)
  line L436 (-10.9, -14) -> (-11.9, -14)
  line L437 (-11.9, -14) -> (-13.9, -12)
  line L438 (-13.9, -12) -> (-13.9, -11)
  line L439 (-13.9, -11) -> (-11.9, -9)
  line L440 (72.2, 11) -> (73.2, 11)
  line L441 (73.2, 11) -> (75.2, 9)
  line L442 (75.2, 9) -> (75.2, 8)
  line L443 (75.2, 8) -> (73.2, 6)
  line L444 (73.2, 6) -> (72.2, 6)
  line L445 (72.2, 6) -> (70.2, 8)
  line L446 (70.2, 8) -> (70.2, 9)
  line L447 (70.2, 9) -> (72.2, 11)
  line L448 (72.2, -9) -> (73.2, -9)
  line L449 (73.2, -9) -> (75.2, -11)
  line L450 (75.2, -11) -> (75.2, -12)
  line L451 (75.2, -12) -> (73.2, -14)
  line L452 (73.2, -14) -> (72.2, -14)
  line L453 (72.2, -14) -> (70.2, -12)
  line L454 (70.2, -12) -> (70.2, -11)
  line L455 (70.2, -11) -> (72.2, -9)
  arc A168 (-108.5929, -2.7071) -> (-107.8858, -3) centre (-107.8858, -2) ccw
  arc A169 (-107.8858, 2) -> (-108.5929, 1.7071) centre (-107.8858, 1) ccw
  line L456 (-108.5929, -2.7071) -> (-110.5, -0.8)
  line L457 (-110.5, -0.5) -> (-110.5, -0.2)
  line L458 (-110.5, -0.5) -> (-110.5, -0.8)
  line L459 (-108.5929, 1.7071) -> (-110.5, -0.2)
  line L460 (-107.8858, 2) -> (-97.1142, 2)
  line L461 (-97.1142, -3) -> (-107.8858, -3)
  arc A170 (-96.4071, 1.7071) -> (-97.1142, 2) centre (-97.1142, 1) ccw
  arc A171 (-97.1142, -3) -> (-96.4071, -2.7071) centre (-97.1142, -2) ccw
  line L462 (-96.4071, -2.7071) -> (-94.5, -0.8)
  line L463 (-94.5, -0.5) -> (-94.5, -0.8)
  line L464 (-94.5, -0.5) -> (-94.5, -0.2)
  line L465 (-96.4071, 1.7071) -> (-94.5, -0.2)
  arc A172 (-109.2929, 2.4071) -> (-109, 3.1142) centre (-110, 3.1142) ccw
  arc A173 (-114, 3.1142) -> (-113.7071, 2.4071) centre (-113, 3.1142) ccw
  line L466 (-109.2929, 2.4071) -> (-111.2, 0.5)
  line L467 (-111.5, 0.5) -> (-111.8, 0.5)
  line L468 (-111.5, 0.5) -> (-111.2, 0.5)
  line L469 (-113.7071, 2.4071) -> (-111.8, 0.5)
  line L470 (-114, 3.1142) -> (-114, 13.8858)
  line L471 (-109, 13.8858) -> (-109, 3.1142)
  arc A174 (-113.7071, 14.5929) -> (-114, 13.8858) centre (-113, 13.8858) ccw
  arc A175 (-109, 13.8858) -> (-109.2929, 14.5929) centre (-110, 13.8858) ccw
  line L472 (-109.2929, 14.5929) -> (-111.2, 16.5)
  line L473 (-111.5, 16.5) -> (-111.2, 16.5)
  line L474 (-111.5, 16.5) -> (-111.8, 16.5)
  line L475 (-113.7071, 14.5929) -> (-111.8, 16.5)
  arc A176 (-126.5929, -2.7071) -> (-125.8858, -3) centre (-125.8858, -2) ccw
  arc A177 (-125.8858, 2) -> (-126.5929, 1.7071) centre (-125.8858, 1) ccw
  line L476 (-126.5929, -2.7071) -> (-128.5, -0.8)
  line L477 (-128.5, -0.5) -> (-128.5, -0.2)
  line L478 (-128.5, -0.5) -> (-128.5, -0.8)
  line L479 (-126.5929, 1.7071) -> (-128.5, -0.2)
  line L480 (-125.8858, 2) -> (-115.1142, 2)
  line L481 (-115.1142, -3) -> (-125.8858, -3)
  arc A178 (-114.4071, 1.7071) -> (-115.1142, 2) centre (-115.1142, 1) ccw
  arc A179 (-115.1142, -3) -> (-114.4071, -2.7071) centre (-115.1142, -2) ccw
  line L482 (-114.4071, -2.7071) -> (-112.5, -0.8)
  line L483 (-112.5, -0.5) -> (-112.5, -0.8)
  line L484 (-112.5, -0.5) -> (-112.5, -0.2)
  line L485 (-114.4071, 1.7071) -> (-112.5, -0.2)
  arc A180 (-109.2929, -15.5929) -> (-109, -14.8858) centre (-110, -14.8858) ccw
  arc A181 (-114, -14.8858) -> (-113.7071, -15.5929) centre (-113, -14.8858) ccw
  line L486 (-109.2929, -15.5929) -> (-111.2, -17.5)
  line L487 (-111.5, -17.5) -> (-111.8, -17.5)
  line L488 (-111.5, -17.5) -> (-111.2, -17.5)
  line L489 (-113.7071, -15.5929) -> (-111.8, -17.5)
  line L490 (-114, -14.8858) -> (-114, -4.1142)
  line L491 (-109, -4.1142) -> (-109, -14.8858)
  arc A182 (-113.7071, -3.4071) -> (-114, -4.1142) centre (-113, -4.1142) ccw
  arc A183 (-109, -4.1142) -> (-109.2929, -3.4071) centre (-110, -4.1142) ccw
  line L492 (-109.2929, -3.4071) -> (-111.2, -1.5)
  line L493 (-111.5, -1.5) -> (-111.2, -1.5)
  line L494 (-111.5, -1.5) -> (-111.8, -1.5)
  line L495 (-113.7071, -3.4071) -> (-111.8, -1.5)
  arc A184 (-138.0929, 13.2929) -> (-137.3858, 13) centre (-137.3858, 14) ccw
  arc A185 (-137.3858, 18) -> (-138.0929, 17.7071) centre (-137.3858, 17) ccw
  line L496 (-138.0929, 13.2929) -> (-140, 15.2)
  line L497 (-140, 15.5) -> (-140, 15.8)
  line L498 (-140, 15.5) -> (-140, 15.2)
  line L499 (-138.0929, 17.7071) -> (-140, 15.8)
  line L500 (-137.3858, 18) -> (-126.6142, 18)
  line L501 (-126.6142, 13) -> (-137.3858, 13)
  arc A186 (-125.9071, 17.7071) -> (-126.6142, 18) centre (-126.6142, 17) ccw
  arc A187 (-126.6142, 13) -> (-125.9071, 13.2929) centre (-126.6142, 14) ccw
  line L502 (-125.9071, 13.2929) -> (-124, 15.2)
  line L503 (-124, 15.5) -> (-124, 15.2)
  line L504 (-124, 15.5) -> (-124, 15.8)
  line L505 (-125.9071, 17.7071) -> (-124, 15.8)
  arc A188 (-155.0929, 13.2929) -> (-154.3858, 13) centre (-154.3858, 14) ccw
  arc A189 (-154.3858, 18) -> (-155.0929, 17.7071) centre (-154.3858, 17) ccw
  line L506 (-155.0929, 13.2929) -> (-157, 15.2)
  line L507 (-157, 15.5) -> (-157, 15.8)
  line L508 (-157, 15.5) -> (-157, 15.2)
  line L509 (-155.0929, 17.7071) -> (-157, 15.8)
  line L510 (-154.3858, 18) -> (-143.6142, 18)
  line L511 (-143.6142, 13) -> (-154.3858, 13)
  arc A190 (-142.9071, 17.7071) -> (-143.6142, 18) centre (-143.6142, 17) ccw
  arc A191 (-143.6142, 13) -> (-142.9071, 13.2929) centre (-143.6142, 14) ccw
  line L512 (-142.9071, 13.2929) -> (-141, 15.2)
  line L513 (-141, 15.5) -> (-141, 15.2)
  line L514 (-141, 15.5) -> (-141, 15.8)
  line L515 (-142.9071, 17.7071) -> (-141, 15.8)
  arc A192 (-138.2929, -0.1071) -> (-138, 0.6) centre (-139, 0.6) ccw
  arc A193 (-143, 0.6) -> (-142.7071, -0.1071) centre (-142, 0.6) ccw
  line L516 (-138.2929, -0.1071) -> (-140.2, -2.0142)
  line L517 (-140.5, -2.0142) -> (-140.8, -2.0142)
  line L518 (-140.5, -2.0142) -> (-140.2, -2.0142)
  line L519 (-142.7071, -0.1071) -> (-140.8, -2.0142)
  line L520 (-143, 0.6) -> (-143, 11.3716)
  line L521 (-138, 11.3716) -> (-138, 0.6)
  arc A194 (-142.7071, 12.0787) -> (-143, 11.3716) centre (-142, 11.3716) ccw
  arc A195 (-138, 11.3716) -> (-138.2929, 12.0787) centre (-139, 11.3716) ccw
  line L522 (-138.2929, 12.0787) -> (-140.2, 13.9858)
  line L523 (-140.5, 13.9858) -> (-140.2, 13.9858)
  line L524 (-140.5, 13.9858) -> (-140.8, 13.9858)
  line L525 (-142.7071, 12.0787) -> (-140.8, 13.9858)
  arc A196 (-138.2929, -17.1071) -> (-138, -16.4) centre (-139, -16.4) ccw
  arc A197 (-143, -16.4) -> (-142.7071, -17.1071) centre (-142, -16.4) ccw
  line L526 (-138.2929, -17.1071) -> (-140.2, -19.0142)
  line L527 (-140.5, -19.0142) -> (-140.8, -19.0142)
  line L528 (-140.5, -19.0142) -> (-140.2, -19.0142)
  line L529 (-142.7071, -17.1071) -> (-140.8, -19.0142)
  line L530 (-143, -16.4) -> (-143, -5.6284)
  line L531 (-138, -5.6284) -> (-138, -16.4)
  arc A198 (-142.7071, -4.9213) -> (-143, -5.6284) centre (-142, -5.6284) ccw
  arc A199 (-138, -5.6284) -> (-138.2929, -4.9213) centre (-139, -5.6284) ccw
  line L532 (-138.2929, -4.9213) -> (-140.2, -3.0142)
  line L533 (-140.5, -3.0142) -> (-140.2, -3.0142)
  line L534 (-140.5, -3.0142) -> (-140.8, -3.0142)
  line L535 (-142.7071, -4.9213) -> (-140.8, -3.0142)
  point P0 (0, 0)
  dimension "d525" = 8
  dimension "d526" = 7.4
  dimension "d527" = 22
  dimension "d528" = 16.7
  dimension "d529" = 8
extrude "Extrusion3" cut sketch "Sketch5" against normal blind 5
sketch "Sketch8" plane through (0, 0, 0) normal (0, 0, -1) x (-1, 0, 0)
  line L0 (-140, 35) -> (140, 35)
  line L1 (165, 10) -> (165, -10)
  line L2 (140, -35) -> (-140, -35)
  line L3 (-165, -10) -> (-165, 10)
  arc A0 (-140, 35) -> (-165, 10) centre (-140, 10) ccw
  arc A1 (165, 10) -> (140, 35) centre (140, 10) ccw
  arc A2 (140, -35) -> (165, -10) centre (140, -10) ccw
  arc A3 (-165, -10) -> (-140, -35) centre (-140, -10) ccw
  point P0 (0, 0)
  dimension "d542" = 35
  dimension "d543" = 165
extrude "Extrusion5" add sketch "Sketch8" along normal blind 3 separate body